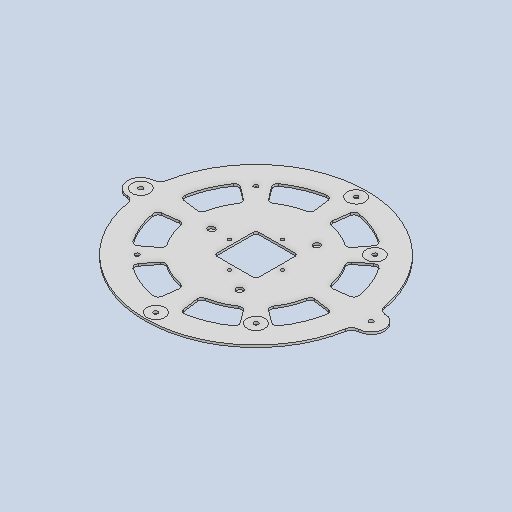
# Autodesk Inventor part: AP-1-02-basePlate
Saved by Autodesk Inventor 2025.1 (Build 291241020, 241B)
## iProperties
Created: 2024-10-16
Part Number: AP-1-02-basePlate
Material: Generic
Document SubType Name: Modeling
Designer: jdl5984
Density: 1 g/cm^3
Appearance: Default
Author: jdl5984
## iProperties of the stored document AP-1-02-basePlate_3DPrint.ipt
Created: 2024-12-05
Part Number: AP-1-02-basePlate_3DPrint
Material: Generic
Document SubType Name: Modeling
Designer: t205b
Density: 1 g/cm^3
Appearance: Default
Author: t205b
Autodesk Inventor part; units mm, degrees
ref_plane "YZ Plane" through (0, 0, 0) normal (1, 0, 0) x (0, 1, 0)
ref_plane "XZ Plane" through (0, 0, 0) normal (0, 1, 0) x (-1, 0, 0)
ref_plane "XY Plane" through (0, 0, 0) normal (0, 0, 1) x (1, 0, 0)
sketch "Sketch1" plane through (0, 0, 0) normal (0, 1, 0) x (-1, 0, 0)
  circle A0 centre (0, 0) radius 158.75
  line L0 (26.05, 30.05) -> (-26.05, 30.05)
  line L1 (-30.05, 26.05) -> (-30.05, -26.05)
  line L2 (-26.05, -30.05) -> (26.05, -30.05)
  line L3 (30.05, -26.05) -> (30.05, 26.05)
  arc A1 (30.05, 26.05) -> (26.05, 30.05) centre (26.05, 26.05) ccw
  arc A2 (26.05, -30.05) -> (30.05, -26.05) centre (26.05, -26.05) ccw
  arc A3 (-30.05, -26.05) -> (-26.05, -30.05) centre (-26.05, -26.05) ccw
  arc A4 (-26.05, 30.05) -> (-30.05, 26.05) centre (-26.05, 26.05) ccw
  circle A5 centre (38, 0) radius 2.5527
  circle A6 centre (0, -38) radius 2.5527
  circle A7 centre (-38, 0) radius 2.5527
  circle A8 centre (0, 38) radius 2.5527
  circle A9 centre (63.909194, 0) radius 4.7625
  circle A10 centre (-31.954597, -55.345443) radius 4.7625
  circle A11 centre (0, 0) radius 63.909194 construction
  circle A12 centre (0, 143.6497) radius 3.20675
  circle A13 centre (0, -143.6497) radius 3.20675
  line L4 (157.602855, 19.05) -> (165.227, 19.05)
  line L5 (165.227, 19.05) -> (165.227, -19.05) construction
  line L6 (165.227, -19.05) -> (157.602855, -19.05)
  line L7 (157.602855, -17.457804) -> (157.602855, 19.05) construction
  arc A14 (165.227, -19.05) -> (165.227, 19.05) centre (165.227, 0) ccw
  circle A15 centre (165.227, 0) radius 3.20675
  line L8 (0, -158.75) -> (0, 158.75) construction
  line L9 (-157.602855, 19.05) -> (-165.227, 19.05)
  line L10 (-165.227, -19.05) -> (-157.602855, -19.05)
  arc A16 (-165.227, 19.05) -> (-165.227, -19.05) centre (-165.227, 0) ccw
  circle A17 centre (-165.227, 0) radius 3.20675
  circle A18 centre (-31.953261, 55.347757) radius 4.7625
  circle A19 centre (-165.227, 0) radius 12.7
  circle A20 centre (165.227, 0) radius 12.7
  point P0 (30.05, 30.05)
  point P1 (-30.05, 30.05)
  point P2 (30.05, -30.05)
  dimension "d84" = 170.6245
  dimension "d0" = 317.5
  dimension "d1" = 30.05
  dimension "d2" = 60.1
  dimension "d3" = 60.1
  dimension "d4" = 30.05
  dimension "d5" = 4
  dimension "d6" = 4
  dimension "d7" = 5.1054
  dimension "d8" = 5.1054
  dimension "d9" = 5.1054
  dimension "d10" = 5.1054
  dimension "d11" = 76
  dimension "d12" = 38
  dimension "d13" = 76
  dimension "d14" = 38
  dimension "d15" = 9.525
  dimension "d17" = 110.6932
  dimension "d20" = 9.525
  dimension "d24" = 6.4135
  dimension "d25" = 6.4135
  dimension "d26" = 287.2994
  dimension "d27" = 143.6497
  dimension "d30" = 38.1
  dimension "d31" = 6.4135
  dimension "d33" = 330.454
  dimension "d38" = 110.6932
  dimension "d39" = 110.6932
  dimension "d41" = 127.81839
  dimension "d141" = 25.4
  dimension "d142" = 25.4
  constraints: 22 end point, 21 centre point, 20 point on circle, 8 tangent, 6 coincident, 6 point on line, 6 symmetric about line, 4 horizontal alignment, 4 parallel, 4 vertical alignment, 3 equal radius, 2 horizontal, 2 perpendicular, 1 midpoint, 1 vertical, 2 other
  measures "d0" diameter of A0
  measures "d1" distance from line of point (0, 0) L3
  measures "d2" distance of point (30.05, 30.05) point (-30.05, 30.05)
  measures "d3" distance of point (30.05, -30.05) point (30.05, 30.05)
  measures "d4" distance from line of point (0, 0) L2
  measures "d5" radius of A1
  measures "d6" radius of A2
  measures "d7" diameter of A5
  measures "d8" diameter of A6
  measures "d9" diameter of A7
  measures "d10" diameter of A8
  measures "d11" distance of A7.centre A5.centre
  measures "d12" distance of point (0, 0) A7.centre
  measures "d13" distance of A8.centre A6.centre
  measures "d14" distance of point (0, 0) A6.centre
  measures "d15" diameter of A9
  measures "d17" distance of A10.centre A9.centre
  measures "d20" diameter of A10
  measures "d24" diameter of A13
  measures "d25" diameter of A12
  measures "d26" distance of A13.centre A12.centre
  measures "d27" distance of A12.centre point (0, 0)
  measures "d30" distance of L4.start L6.end
  measures "d31" diameter of A15
  measures "d33" distance of A17.centre A14.centre
  measures "d38" distance of A18.centre A10.centre
  measures "d39" distance of A9.centre A18.centre
  measures "d41" diameter of A11
  measures "d141" diameter of A19
  measures "d142" diameter of A20
extrude "Extrusion1" add sketch "Sketch1" along normal blind 3.175
fillet "Fillet1" radius 10.16 4 edges at (-157.6029, 1.5875, 19.05) (-157.6029, 1.5875, -19.05) (157.6029, 1.5875, -19.05) (157.6029, 1.5875, 19.05)
sketch "Sketch4" plane through (0, 3.175, 0) normal (0, 1, 0) x (1, 0, 0)
  circle A0 centre (-85.31225, 85.31225) radius 3.175
  circle A1 centre (85.31225, 85.312983) radius 3.175
  circle A2 centre (85.31225, -85.312983) radius 3.175
  circle A3 centre (-85.31225, -85.31225) radius 3.175
  point P0 (0, 0)
  dimension "d79" = 6.35
  dimension "d80" = 6.35
  dimension "d81" = 6.35
  dimension "d82" = 6.35
  dimension "d83" = 241.3
  dimension "d84" = 170.6245
  dimension "d85" = 170.6245
  dimension "d86" = 241.3
  dimension "d94" = 85.31225
  dimension "d95" = 85.31225
  constraints: 4 centre point, 2 vertical alignment
  measures "d79" diameter of A0
  measures "d80" diameter of A1
  measures "d81" diameter of A2
  measures "d82" diameter of A3
  measures "d83" distance of A2.centre A0.centre
  measures "d84" distance of A3.centre A0.centre
  measures "d85" distance of A1.centre A0.centre
  measures "d86" distance of A3.centre A1.centre
  measures "d94" horizontal distance of A2.centre point (0, 0)
  measures "d95" horizontal distance of point (0, 0) A3.centre
extrude "Extrusion3" cut sketch "Sketch4" against normal blind 6.35
sketch "Sketch2" plane through (0, 3.175, 0) normal (0, 1, 0) x (1, 0, 0)
  circle A0 centre (0, 0) radius 127
  circle A1 centre (0, 0) radius 92.075
  line L0 (-56.051709, 73.048009) -> (-77.312701, 100.755874)
  line L1 (-73.048009, 56.051709) -> (-100.755874, 77.312701)
  line L2 (0, -163.129758) -> (0, 179.038142) construction
  line L3 (-207.242994, 0) -> (231.197684, 0) construction
  arc A2 (156.36191, 27.432016) -> (-156.36191, 27.432016) centre (0, 0) ccw
  line L4 (-91.287286, 12.018199) -> (-125.913497, 16.576826)
  line L5 (-91.287286, -12.018199) -> (-125.913497, -16.576826)
  line L6 (-73.048009, -56.051709) -> (-100.755874, -77.312701)
  line L7 (-56.051709, -73.048009) -> (-77.312701, -100.755874)
  line L8 (-12.018199, -91.287286) -> (-16.576826, -125.913497)
  line L9 (12.018199, -91.287286) -> (16.576826, -125.913497)
  line L10 (56.051709, -73.048009) -> (77.312701, -100.755874)
  line L11 (73.048009, -56.051709) -> (100.755874, -77.312701)
  line L12 (91.287286, -12.018199) -> (125.913497, -16.576826)
  line L13 (91.287286, 12.018199) -> (125.913497, 16.576826)
  line L14 (73.048009, 56.051709) -> (100.755874, 77.312701)
  line L15 (56.051709, 73.048009) -> (77.312701, 100.755874)
  line L16 (12.018199, 91.287286) -> (16.576826, 125.913497)
  line L17 (-12.018199, 91.287286) -> (-16.576826, 125.913497)
  dimension "d96" = 254
  dimension "d97" = 184.15
  dimension "d98" = 15
  dimension "d99" = 37.5
  dimension "d102" = 360
  constraints: 36 end point, 4 line through centre, 4 point on circle, 2 centre point, 2 coincident, 1 concentric, 1 horizontal, 1 vertical, 49 other
  measures "d96" diameter of A0
  measures "d97" diameter of A1
  measures "d98" angle of L1 L0
  measures "d99" angle of L2 L0
extrude "Extrusion2" cut sketch "Sketch2" against normal blind 6.35 contours L13 A1 L14 A0 | A0 L11 A1 L12 | L15 A1 L16 A0 | A0 L9 A1 L10 | L17 A1 L0 A0 | A0 L7 A1 L8 | L1 A1 L4 A0 | A0 L5 A1 L6
fillet "Fillet5" radius 6.35 32 edges at (77.3127, 1.5875, -100.7559) (100.7559, 1.5875, -77.3127) (73.048, 1.5875, -56.0517) (56.0517, 1.5875, -73.048) (91.2873, 1.5875, -12.0182) (125.9135, 1.5875, -16.5768) (125.9135, 1.5875, 16.5768) (91.2873, 1.5875, 12.0182) (100.7559, 1.5875, 77.3127) (73.048, 1.5875, 56.0517) (56.0517, 1.5875, 73.048) (12.0182, 1.5875, 91.2873) (16.5768, 1.5875, 125.9135) (77.3127, 1.5875, 100.7559) (-16.5768, 1.5875, 125.9135) (-12.0182, 1.5875, 91.2873) (-56.0517, 1.5875, 73.048) (-77.3127, 1.5875, 100.7559) (-100.7559, 1.5875, 77.3127) (-73.048, 1.5875, 56.0517) (-91.2873, 1.5875, 12.0182) (-125.9135, 1.5875, 16.5768) (-91.2873, 1.5875, -12.0182) (-125.9135, 1.5875, -16.5768) (-100.7559, 1.5875, -77.3127) (-73.048, 1.5875, -56.0517) (16.5768, 1.5875, -125.9135) (12.0182, 1.5875, -91.2873) (-12.0182, 1.5875, -91.2873) (-16.5768, 1.5875, -125.9135) (-77.3127, 1.5875, -100.7559) (-56.0517, 1.5875, -73.048)
sketch "Sketch5" plane through (0, 3.175, 0) normal (0, 1, 0) x (1, 0, 0)
  arc A0 (156.36191, 27.432016) -> (-156.36191, 27.432016) centre (0, 0) ccw
  line L0 (114.323629, 93.503259) -> (107.746808, 85.609658)
  line L1 (102.794876, 85.701097) -> (98.942848, 90.687775)
  line L2 (96.430198, 91.921844) -> (82.642149, 91.921844)
  line L3 (79.820984, 90.203432) -> (62.926749, 57.482159)
  line L4 (58.073213, 56.499466) -> (54.345012, 59.605743)
  line L5 (49.539533, 58.712583) -> (43.644939, 48.140102)
  line L6 (45.733493, 43.493655) -> (54.672045, 41.520015)
  line L7 (55.928422, 35.907041) -> (38.396768, 22.364472)
  line L8 (36.455837, 21.702122) -> (30.05, 21.702122)
  arc A1 (114.323629, 93.503259) -> (114.08506, 97.824185) centre (111.884347, 95.53563) ccw
  arc A2 (102.794876, 85.701097) -> (107.746808, 85.609658) centre (105.307526, 87.642029) ccw
  arc A3 (98.942848, 90.687775) -> (96.430198, 91.921844) centre (96.430198, 88.746844) ccw
  arc A4 (82.642149, 91.921844) -> (79.820984, 90.203432) centre (82.642149, 88.746844) ccw
  arc A5 (58.073213, 56.499466) -> (62.926749, 57.482159) centre (60.105584, 58.938747) ccw
  arc A6 (54.345012, 59.605743) -> (49.539533, 58.712583) centre (52.312642, 57.166461) ccw
  arc A7 (43.644939, 48.140102) -> (45.733493, 43.493655) centre (46.418047, 46.59398) ccw
  arc A8 (55.928422, 35.907041) -> (54.672045, 41.520015) centre (53.98749, 38.419691) ccw
  arc A9 (36.455837, 21.702122) -> (38.396768, 22.364472) centre (36.455837, 24.877122) ccw
  line L9 (30.05, 26.05) -> (30.05, -26.05)
  line L10 (-117.684254, 106.545665) -> (-111.690373, 95.877786)
  line L11 (-117.684254, 106.545665) -> (-105.447823, 106.545665) construction
  line L12 (-106.314926, 95.62143) -> (-100.095577, 104.572983)
  line L13 (-95.210356, 104.973253) -> (-73.802538, 82.927472)
  line L14 (-74.525079, 77.947601) -> (-78.919769, 75.47839)
  line L15 (-78.664082, 69.813526) -> (-51.960748, 57.834208)
  line L16 (-47.486196, 60.731067) -> (-47.486196, 61.336583)
  line L17 (-44.745097, 64.481794) -> (-25.696601, 67.109654)
  line L18 (-22.146625, 64.573297) -> (-15.401069, 30.05)
  line L19 (-26.05, 30.05) -> (26.05, 30.05)
  arc A10 (-111.690373, 95.877786) -> (-106.314926, 95.62143) centre (-108.922367, 97.433025) ccw
  arc A11 (-95.210356, 104.973253) -> (-100.095577, 104.572983) centre (-97.488136, 102.761389) ccw
  arc A12 (-74.525079, 77.947601) -> (-73.802538, 82.927472) centre (-76.080318, 80.715607) ccw
  arc A13 (-78.919769, 75.47839) -> (-78.664082, 69.813526) centre (-77.36453, 72.710384) ccw
  arc A14 (-51.960748, 57.834208) -> (-47.486196, 60.731067) centre (-50.661196, 60.731067) ccw
  arc A15 (-22.146625, 64.573297) -> (-25.696601, 67.109654) centre (-25.2627, 63.964442) ccw
  arc A16 (-44.745097, 64.481794) -> (-47.486196, 61.336583) centre (-44.311196, 61.336583) ccw
  arc A17 (-156.36191, -27.432016) -> (156.36191, -27.432016) centre (0, 0) ccw
  line L20 (119.756418, -104.211145) -> (114.197701, -94.483027)
  line L21 (109.920807, -93.270819) -> (97.333567, -100.135661)
  line L22 (93.792155, -99.79679) -> (75.124201, -84.386778)
  line L23 (76.230235, -78.898002) -> (76.783348, -78.731503)
  line L24 (76.889993, -72.685184) -> (51.417633, -64.026624)
  line L25 (49.668867, -59.469918) -> (57.624815, -45.254613)
  line L26 (53.334027, -40.916578) -> (42.26298, -46.954517)
  line L27 (39.993091, -47.252333) -> (30.826695, -45.024951)
  line L28 (29.558719, -33.370158) -> (19.931137, -30.05)
  line L29 (26.05, -30.05) -> (-26.05, -30.05)
  arc A18 (30.05, -39.155709) -> (29.558719, -33.370158) centre (28.523614, -36.371688) ccw
  arc A19 (30.05, -39.155709) -> (30.826695, -45.024951) centre (31.576386, -41.93973) ccw
  arc A20 (39.993091, -47.252333) -> (42.26298, -46.954517) centre (40.742782, -44.167112) ccw
  arc A21 (57.624815, -45.254613) -> (53.334027, -40.916578) centre (54.854224, -43.703983) ccw
  arc A22 (49.668867, -59.469918) -> (51.417633, -64.026624) centre (52.439458, -61.020547) ccw
  arc A23 (76.783348, -78.731503) -> (76.889993, -72.685184) centre (75.868167, -75.691261) ccw
  arc A24 (76.230235, -78.898002) -> (75.124201, -84.386778) centre (77.145415, -81.938244) ccw
  arc A25 (93.792155, -99.79679) -> (97.333567, -100.135661) centre (95.81337, -97.348256) ccw
  arc A26 (114.197701, -94.483027) -> (109.920807, -93.270819) centre (111.441004, -96.058224) ccw
  line L30 (-104.978812, -99.339676) -> (-112.161366, -95.757781)
  line L31 (-112.232195, -90.111641) -> (-82.888145, -74.546819)
  line L32 (-78.374865, -76.388926) -> (-76.351209, -82.74846)
  line L33 (-70.15342, -81.917287) -> (-68.70325, -46.952579)
  line L34 (-68.790877, -46.068957) -> (-70.602028, -38.640259)
  line L35 (-66.815629, -34.791731) -> (-52.196463, -38.104865)
  line L36 (-48.410064, -34.256337) -> (-51.914184, -19.883685)
  line L37 (-50.197881, -16.266628) -> (-30.05, -6.643883)
  line L38 (-30.05, -26.05) -> (-30.05, 26.05)
  arc A27 (-50.197881, -16.266628) -> (-51.914184, -19.883685) centre (-48.829538, -19.131634) ccw
  arc A28 (-52.196463, -38.104865) -> (-48.410064, -34.256337) centre (-51.494711, -35.008388) ccw
  arc A29 (-66.815629, -34.791731) -> (-70.602028, -38.640259) centre (-67.517382, -37.888208) ccw
  arc A30 (-68.70325, -46.952579) -> (-68.790877, -46.068957) centre (-71.875523, -46.821009) ccw
  arc A31 (-76.351209, -82.74846) -> (-70.15342, -81.917287) centre (-73.325693, -81.785716) ccw
  arc A32 (-78.374865, -76.388926) -> (-82.888145, -74.546819) centre (-81.400382, -77.35167) ccw
  arc A33 (-112.232195, -90.111641) -> (-112.161366, -95.757781) centre (-110.744432, -92.916492) ccw
  arc A34 (-106.067701, -105.338973) -> (-104.978812, -99.339676) centre (-106.395746, -102.180966) ccw
  line L39 (-106.067701, -105.338973) -> (-117.684254, -106.545665)
  line L40 (-15.401069, 30.05) -> (-30.05, -6.643883)
  line L41 (30.05, 21.702122) -> (19.931137, -30.05)
  arc A35 (113.168341, 100.714603) -> (114.08506, 97.824185) centre (116.285773, 100.112741) ccw
  line L42 (113.168341, 100.714603) -> (114.87728, 109.566295)
  point P0 (-30.05, -6.643883)
  point P1 (-59.506046, -36.448298)
  point P2 (-65.312415, 63.823867)
  dimension "d107" = 3.175
  dimension "d108" = 3.175
  dimension "d109" = 3.175
  dimension "d119" = 11.61655
  dimension "d120" = 10.57248
  dimension "d121" = 8.93855
  dimension "d122" = 16.89423
  dimension "d123" = 9.62758
  dimension "d124" = 5.55872
  dimension "d125" = 9.72812
  dimension "d126" = 18.66795
  dimension "d127" = 13.54257
  dimension "d128" = 6.40584
  dimension "d129" = 8.34788
  dimension "d130" = 0.55311
  dimension "d131" = 3.175
  dimension "d132" = 8.85169
  dimension "d133" = 1.97364
  constraints: 78 end point, 74 point on circle, 65 tangent, 34 centre point, 30 equal radius, 8 point on line, 3 horizontal, 3 parallel, 3 perpendicular, 2 midpoint, 1 equal length, 1 vertical, 28 other
  measures "d107" radius of A10
  measures "d108" radius of A18
  measures "d109" radius of A27
  measures "d119" horizontal distance of L39.start L39.end
  measures "d120" vertical distance of L5.start L5.end
  measures "d121" horizontal distance of L6.start L6.end
  measures "d122" horizontal distance of L3.start L3.end
  measures "d123" horizontal distance of L28.start L28.end
  measures "d124" horizontal distance of L20.start L20.end
  measures "d125" vertical distance of L20.start L20.end
  measures "d126" horizontal distance of L22.start L22.end
  measures "d127" vertical distance of L7.start L7.end
  measures "d128" distance of L8.start L8.end
  measures "d129" distance between parallel lines of L19 L8
  measures "d130" horizontal distance of L23.start L23.end
  measures "d131" radius of A35
  measures "d132" vertical distance of L42.start L42.end
  measures "d133" vertical distance of L6.start L6.end
split "Split17" [suppressed]
split "Split18" [suppressed]
sketch "Sketch6" plane through (0, 3.175, 0) normal (0, 1, 0) x (1, 0, 0)
  line L0 (26.724656, 0) -> (-26.850041, 0)
  line L1 (-30.05, -6.643883) -> (-30.05, 26.05)
  point P0 (0, 0)
  constraints: 2 end point, 1 perpendicular
split "Split19" [suppressed]
sketch "Sketch8" plane through (0, 3.175, 0) normal (0, 1, 0) x (1, 0, 0)
  circle A0 centre (85.31225, 85.312983) radius 3.175
  circle A1 centre (85.31225, 85.312983) radius 12.7
  circle A2 centre (85.31225, -85.312983) radius 3.175
  circle A3 centre (85.31225, -85.312983) radius 12.7
  circle A4 centre (-165.227, 0) radius 3.20675
  circle A5 centre (-165.227, 0) radius 12.7
  circle A6 centre (0, -143.6497) radius 3.20675
  circle A7 centre (0, -143.6497) radius 12.7
  circle A8 centre (0, 143.6497) radius 3.20675
  circle A9 centre (0, 143.6497) radius 12.7
  point P0 (0, 0)
  dimension "d135" = 25.4
  dimension "d136" = 25.4
  dimension "d137" = 25.4
  dimension "d147" = 25.4
  dimension "d148" = 25.4
  constraints: 5 centre point, 5 coincident
  measures "d135" diameter of A1
  measures "d136" diameter of A3
  measures "d137" diameter of A5
  measures "d147" diameter of A7
  measures "d148" diameter of A9
sketch "Sketch9" plane through (0, 0, 0) normal (0, -1, 0) x (1, 0, 0)
  circle A0 centre (-85.31225, 85.31225) radius 3.175
  circle A1 centre (-85.31225, 85.31225) radius 12.7
  circle A2 centre (-85.31225, -85.31225) radius 3.175
  circle A3 centre (-85.31225, -85.31225) radius 12.7
  circle A4 centre (165.227, 0) radius 3.20675
  circle A5 centre (165.227, 0) radius 12.7
  circle A6 centre (0, -143.6497) radius 3.20675
  circle A7 centre (0, -143.6497) radius 12.7
  circle A8 centre (0, 143.6497) radius 3.20675
  circle A9 centre (0, 143.6497) radius 12.7
  point P0 (0, 0)
  dimension "d138" = 25.4
  dimension "d139" = 25.4
  dimension "d140" = 25.4
  dimension "d149" = 25.4
  dimension "d150" = 25.4
  constraints: 5 centre point, 5 coincident
  measures "d138" diameter of A1
  measures "d139" diameter of A3
  measures "d140" diameter of A5
  measures "d149" diameter of A7
  measures "d150" diameter of A9
extrude "Extrusion4" add sketch "Sketch8" along normal blind 0.000025
extrude "Extrusion5" add sketch "Sketch9" along normal blind 0.000025
equation "\"d24\" = d25"
equation "\"d25\" = d31"
equation "\"d38\" = d17"
equation "\"d39\" = d17"
body "Solid1"
body "Solid34"
body "Solid35"
body "Solid38"
body "Solid39"
body "Solid40"
body "Solid41"
